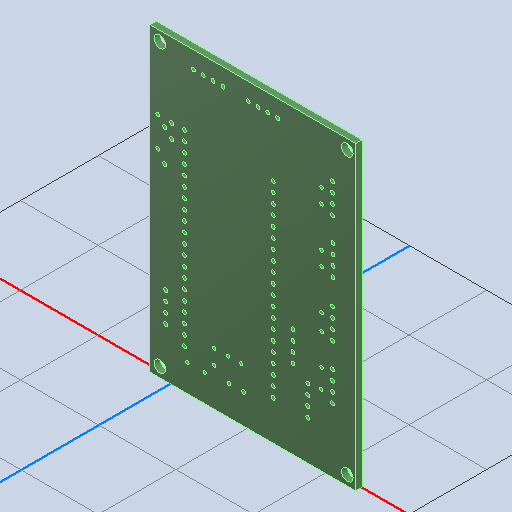
# Autodesk Inventor part: main_pcb.brd
Saved by Autodesk Inventor 2022 (Build 260153000, 153)
## iProperties
Created: 2021-08-05
Part Number: main_pcb.brd
Material: Типовые
Document SubType Name: Modeling
Designer: Петров Иван
Mass: 6.40297 g
Surface Area: 89.7072 cm^2
Volume: 6.40297 cm^3
Density: 1 g/cm^3
Appearance: Контур панели
Author: Петров Иван
Autodesk Inventor part; units mm, degrees
ref_plane "YZ Plane" through (0, 0, 0) normal (1, 0, 0) x (0, 1, 0)
ref_plane "XZ Plane" through (0, 0, 0) normal (0, 1, 0) x (-1, 0, 0)
ref_plane "XY Plane" through (0, 0, 0) normal (0, 0, 1) x (1, 0, 0)
sketch "Эскиз1" plane through (0, 0, 0) normal (0, 0, 1) x (1, 0, 0)
  line L0 (-5.08, 0) -> (47.93, 0)
  line L1 (47.93, 0) -> (47.93, 77.46)
  line L2 (47.93, 77.46) -> (-5.08, 77.46)
  line L3 (-5.08, 77.46) -> (-5.08, 0)
  circle A0 centre (41.91, 66.04) radius 0.51
  circle A1 centre (41.91, 63.5) radius 0.51
  circle A2 centre (41.91, 60.96) radius 0.51
  circle A3 centre (41.91, 58.42) radius 0.51
  circle A4 centre (42.04, 52.32) radius 0.51
  circle A5 centre (42.04, 49.78) radius 0.51
  circle A6 centre (42.04, 47.24) radius 0.51
  circle A7 centre (42.04, 44.7) radius 0.51
  circle A8 centre (41.91, 38.1) radius 0.51
  circle A9 centre (41.91, 35.56) radius 0.51
  circle A10 centre (41.91, 33.02) radius 0.51
  circle A11 centre (41.91, 30.48) radius 0.51
  circle A12 centre (41.91, 24.13) radius 0.51
  circle A13 centre (41.91, 21.59) radius 0.51
  circle A14 centre (41.91, 19.05) radius 0.51
  circle A15 centre (41.91, 16.51) radius 0.51
  circle A16 centre (13.72, 73.03) radius 0.51
  circle A17 centre (11.18, 73.03) radius 0.51
  circle A18 centre (8.64, 73.03) radius 0.51
  circle A19 centre (6.1, 73.03) radius 0.51
  circle A20 centre (27.81, 73.03) radius 0.51
  circle A21 centre (25.27, 73.03) radius 0.51
  circle A22 centre (22.73, 73.03) radius 0.51
  circle A23 centre (20.19, 73.03) radius 0.51
  circle A24 centre (35.56, 17.78) radius 0.51
  circle A25 centre (35.56, 15.24) radius 0.51
  circle A26 centre (35.56, 12.7) radius 0.51
  circle A27 centre (35.56, 10.16) radius 0.51
  circle A28 centre (-1.02, 12.7) radius 0.51
  circle A29 centre (-1.02, 15.24) radius 0.51
  circle A30 centre (-1.02, 17.78) radius 0.51
  circle A31 centre (-1.02, 20.32) radius 0.51
  circle A32 centre (31.75, 27.94) radius 0.51
  circle A33 centre (31.75, 25.4) radius 0.51
  circle A34 centre (31.75, 22.86) radius 0.51
  circle A35 centre (31.75, 20.32) radius 0.51
  circle A36 centre (-3.05, 50.8) radius 0.5
  circle A37 centre (-3.05, 58.42) radius 0.5
  circle A38 centre (0.51, 58.31) radius 0.5
  circle A39 centre (-1.29, 56.52) radius 0.5
  circle A40 centre (0.51, 54.72) radius 0.5
  circle A41 centre (3.81, 48.26) radius 0.5
  circle A42 centre (3.81, 45.72) radius 0.5
  circle A43 centre (3.81, 43.18) radius 0.5
  circle A44 centre (3.81, 40.64) radius 0.5
  circle A45 centre (3.81, 53.34) radius 0.5
  circle A46 centre (3.81, 38.1) radius 0.5
  circle A47 centre (3.81, 35.56) radius 0.5
  circle A48 centre (3.81, 55.88) radius 0.5
  circle A49 centre (26.67, 12.7) radius 0.5
  circle A50 centre (3.81, 33.02) radius 0.5
  circle A51 centre (3.81, 30.48) radius 0.5
  circle A52 centre (3.81, 27.94) radius 0.5
  circle A53 centre (3.81, 25.4) radius 0.5
  circle A54 centre (3.81, 22.86) radius 0.5
  circle A55 centre (3.81, 20.32) radius 0.5
  circle A56 centre (3.81, 17.78) radius 0.5
  circle A57 centre (3.81, 15.24) radius 0.5
  circle A58 centre (3.81, 12.7) radius 0.5
  circle A59 centre (3.81, 10.16) radius 0.5
  circle A60 centre (26.67, 38.1) radius 0.5
  circle A61 centre (26.67, 35.56) radius 0.5
  circle A62 centre (26.67, 33.02) radius 0.5
  circle A63 centre (26.67, 30.48) radius 0.5
  circle A64 centre (26.67, 27.94) radius 0.5
  circle A65 centre (26.67, 25.4) radius 0.5
  circle A66 centre (26.67, 22.86) radius 0.5
  circle A67 centre (26.67, 20.32) radius 0.5
  circle A68 centre (26.67, 17.78) radius 0.5
  circle A69 centre (26.67, 15.24) radius 0.5
  circle A70 centre (26.67, 10.16) radius 0.5
  circle A71 centre (26.67, 45.72) radius 0.5
  circle A72 centre (3.81, 50.8) radius 0.5
  circle A73 centre (26.67, 53.34) radius 0.5
  circle A74 centre (26.67, 50.8) radius 0.5
  circle A75 centre (26.67, 40.64) radius 0.5
  circle A76 centre (3.81, 58.42) radius 0.5
  circle A77 centre (26.67, 48.26) radius 0.5
  circle A78 centre (26.67, 58.42) radius 0.5
  circle A79 centre (26.67, 55.88) radius 0.5
  circle A80 centre (26.67, 43.18) radius 0.5
  circle A81 centre (-2.54, 74.93) radius 1.5
  circle A82 centre (45.72, 74.93) radius 1.5
  circle A83 centre (45.72, 2.54) radius 1.5
  circle A84 centre (-2.54, 2.54) radius 1.5
  circle A85 centre (19.05, 7.62) radius 0.5
  circle A86 centre (39.116, 63.246) radius 0.45
  circle A87 centre (39.116, 59.563) radius 0.45
  circle A88 centre (39.116, 49.276) radius 0.45
  circle A89 centre (39.116, 45.593) radius 0.45
  circle A90 centre (39.116, 35.306) radius 0.45
  circle A91 centre (39.116, 31.115) radius 0.45
  circle A92 centre (39.116, 23.114) radius 0.45
  circle A93 centre (38.989, 18.161) radius 0.45
  circle A94 centre (14.986, 13.589) radius 0.45
  circle A95 centre (18.415, 13.589) radius 0.45
  circle A96 centre (11.43, 13.589) radius 0.45
  circle A97 centre (11.43, 9.779) radius 0.45
  circle A98 centre (4.572, 6.985) radius 0.45
  circle A99 centre (9.017, 6.985) radius 0.45
  circle A100 centre (15.24, 7.62) radius 0.5
  circle A101 centre (-1.27, 48.26) radius 0.5
  constraints: 102 centre point, 8 end point
extrude "main_pcb.brdКонтур" add sketch "Эскиз1" along normal blind 1.6
